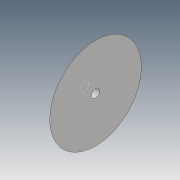
# Autodesk Inventor part: Piatto
Saved by Autodesk Inventor 2018 (Build 220112000, 112)
## iProperties
Created: 2019-02-28
Part Number: Piatto
Material: Generic
Document SubType Name: Modeling
Designer: lutepd0
Density: 1 g/cm^3
Appearance: Default
Author: lutepd0
Autodesk Inventor part; units mm, degrees
ref_plane "YZ Plane" through (0, 0, 0) normal (1, 0, 0) x (0, 1, 0)
ref_plane "XZ Plane" through (0, 0, 0) normal (0, 1, 0) x (-1, 0, 0)
ref_plane "XY Plane" through (0, 0, 0) normal (0, 0, 1) x (1, 0, 0)
sketch "Schizzo2" plane through (0, 0, 0) normal (0, 1, 0) x (-1, 0, 0)
  line L0 (0, 0) -> (0, -100)
  line L1 (0, -100) -> (26.7949, 0)
  line L2 (49.1742, 10) -> (-11.2229, 10) construction
  line L3 (0, 0) -> (26.7949, 0)
  dimension "d4" = 100
  dimension "d5" = 15
  dimension "d7" = 10
  constraints: 8 end point, 2 horizontal, 1 vertical
  measures "d4" distance of L0.start L0.end
  measures "d5" angle of L0 L1
  measures "d7" distance between parallel lines of L2 L3
revolve "Rivoluzione4" add sketch "Schizzo2" angle 360 about axis through (-49.1742, 0, 10) along (1, 0, 0)
